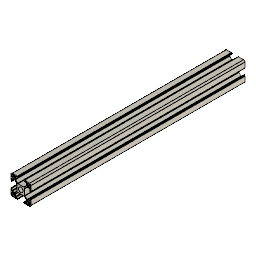
3030_Extrusion_Y_F01 (Autodesk Fusion 360 design; units mm, degrees)
Autodesk Fusion 360 part; units mm, degrees
sketch "スケッチ1" plane through (0, 0, 0) normal (0, 1, 0) x (1, 0, 0)
  line L0 (13, -15) -> (-13, -15)
  line L1 (-15, -13) -> (-15, 13)
  line L2 (-13, 15) -> (13, 15)
  line L3 (15, 13) -> (15, -13)
  line L4 (15, -15) -> (-15, 15) construction
  line L5 (-15, -15) -> (15, 15) construction
  circle A0 centre (0, 0) radius 3.4
  line L6 (-5.2, -15) -> (-5.2, -14.25)
  line L7 (-5.2, -14.25) -> (-4.2, -14.25)
  line L8 (-4.2, -14.25) -> (-4.2, -13.5)
  line L9 (-4.2, -13.5) -> (-7.75, -13.5)
  line L10 (-8.25, -13) -> (-8.25, -9.5178)
  line L11 (-8.1036, -9.1642) -> (-4.8858, -5.9464)
  line L12 (-4.5322, -5.8) -> (0, -5.8)
  arc A1 (-8.25, -13) -> (-7.75, -13.5) centre (-7.75, -13) ccw
  arc A2 (-8.1036, -9.1642) -> (-8.25, -9.5178) centre (-7.75, -9.5178) ccw
  arc A3 (-4.5322, -5.8) -> (-4.8858, -5.9464) centre (-4.5322, -6.3) ccw
  line L13 (-13, -13.5) -> (-10, -13.5)
  line L14 (-9.5, -13) -> (-9.5, -10)
  line L15 (-10, -9.5) -> (-13, -9.5)
  line L16 (-13.5, -10) -> (-13.5, -13)
  arc A4 (-13.5, -13) -> (-13, -13.5) centre (-13, -13) ccw
  arc A5 (-10, -13.5) -> (-9.5, -13) centre (-10, -13) ccw
  arc A6 (-9.5, -10) -> (-10, -9.5) centre (-10, -10) ccw
  arc A7 (-13, -9.5) -> (-13.5, -10) centre (-13, -10) ccw
  arc A8 (-15, -13) -> (-13, -15) centre (-13, -13) ccw
  arc A9 (-13, 15) -> (-15, 13) centre (-13, 13) ccw
  arc A10 (15, 13) -> (13, 15) centre (13, 13) ccw
  arc A11 (13, -15) -> (15, -13) centre (13, -13) ccw
  line L17 (0, 0) -> (0, -15) construction
  line L18 (5.2, -15) -> (5.2, -14.25)
  line L19 (5.2, -14.25) -> (4.2, -14.25)
  line L20 (4.2, -14.25) -> (4.2, -13.5)
  line L21 (4.2, -13.5) -> (7.75, -13.5)
  arc A12 (7.75, -13.5) -> (8.25, -13) centre (7.75, -13) ccw
  line L22 (8.25, -13) -> (8.25, -9.5178)
  arc A13 (8.25, -9.5178) -> (8.1036, -9.1642) centre (7.75, -9.5178) ccw
  line L23 (8.1036, -9.1642) -> (4.8858, -5.9464)
  arc A14 (4.8858, -5.9464) -> (4.5322, -5.8) centre (4.5322, -6.3) ccw
  line L24 (4.5322, -5.8) -> (0, -5.8)
  line L25 (15, -5.2) -> (14.25, -5.2)
  line L26 (14.25, -5.2) -> (14.25, -4.2)
  line L27 (14.25, -4.2) -> (13.5, -4.2)
  line L28 (13.5, -4.2) -> (13.5, -7.75)
  arc A15 (13, -8.25) -> (13.5, -7.75) centre (13, -7.75) ccw
  line L29 (13, -8.25) -> (9.5178, -8.25)
  arc A16 (9.1642, -8.1036) -> (9.5178, -8.25) centre (9.5178, -7.75) ccw
  line L30 (9.1642, -8.1036) -> (5.9464, -4.8858)
  arc A17 (5.8, -4.5322) -> (5.9464, -4.8858) centre (6.3, -4.5322) ccw
  line L31 (5.8, -4.5322) -> (5.8, 0)
  line L32 (5.8, 4.5322) -> (5.8, 0)
  arc A18 (5.9464, 4.8858) -> (5.8, 4.5322) centre (6.3, 4.5322) ccw
  line L33 (9.1642, 8.1036) -> (5.9464, 4.8858)
  arc A19 (9.5178, 8.25) -> (9.1642, 8.1036) centre (9.5178, 7.75) ccw
  line L34 (13, 8.25) -> (9.5178, 8.25)
  arc A20 (13.5, 7.75) -> (13, 8.25) centre (13, 7.75) ccw
  line L35 (13.5, 4.2) -> (13.5, 7.75)
  line L36 (14.25, 4.2) -> (13.5, 4.2)
  line L37 (14.25, 5.2) -> (14.25, 4.2)
  line L38 (15, 5.2) -> (14.25, 5.2)
  line L39 (13.5, -13) -> (13.5, -10)
  arc A21 (13.5, -10) -> (13, -9.5) centre (13, -10) ccw
  line L40 (13, -9.5) -> (10, -9.5)
  arc A22 (10, -9.5) -> (9.5, -10) centre (10, -10) ccw
  line L41 (9.5, -10) -> (9.5, -13)
  arc A23 (9.5, -13) -> (10, -13.5) centre (10, -13) ccw
  line L42 (10, -13.5) -> (13, -13.5)
  arc A24 (13, -13.5) -> (13.5, -13) centre (13, -13) ccw
  line L43 (5.2, 15) -> (5.2, 14.25)
  line L44 (5.2, 14.25) -> (4.2, 14.25)
  line L45 (4.2, 14.25) -> (4.2, 13.5)
  line L46 (4.2, 13.5) -> (7.75, 13.5)
  arc A25 (8.25, 13) -> (7.75, 13.5) centre (7.75, 13) ccw
  line L47 (8.25, 13) -> (8.25, 9.5178)
  arc A26 (8.1036, 9.1642) -> (8.25, 9.5178) centre (7.75, 9.5178) ccw
  line L48 (8.1036, 9.1642) -> (4.8858, 5.9464)
  arc A27 (4.5322, 5.8) -> (4.8858, 5.9464) centre (4.5322, 6.3) ccw
  line L49 (4.5322, 5.8) -> (0, 5.8)
  line L50 (-4.5322, 5.8) -> (0, 5.8)
  arc A28 (-4.8858, 5.9464) -> (-4.5322, 5.8) centre (-4.5322, 6.3) ccw
  line L51 (-8.1036, 9.1642) -> (-4.8858, 5.9464)
  arc A29 (-8.25, 9.5178) -> (-8.1036, 9.1642) centre (-7.75, 9.5178) ccw
  line L52 (-8.25, 13) -> (-8.25, 9.5178)
  arc A30 (-7.75, 13.5) -> (-8.25, 13) centre (-7.75, 13) ccw
  line L53 (-4.2, 13.5) -> (-7.75, 13.5)
  line L54 (-4.2, 14.25) -> (-4.2, 13.5)
  line L55 (-5.2, 14.25) -> (-4.2, 14.25)
  line L56 (-5.2, 15) -> (-5.2, 14.25)
  line L57 (13, 13.5) -> (10, 13.5)
  arc A31 (10, 13.5) -> (9.5, 13) centre (10, 13) ccw
  line L58 (9.5, 13) -> (9.5, 10)
  arc A32 (9.5, 10) -> (10, 9.5) centre (10, 10) ccw
  line L59 (10, 9.5) -> (13, 9.5)
  arc A33 (13, 9.5) -> (13.5, 10) centre (13, 10) ccw
  line L60 (13.5, 10) -> (13.5, 13)
  arc A34 (13.5, 13) -> (13, 13.5) centre (13, 13) ccw
  line L61 (-15, 5.2) -> (-14.25, 5.2)
  line L62 (-14.25, 5.2) -> (-14.25, 4.2)
  line L63 (-14.25, 4.2) -> (-13.5, 4.2)
  line L64 (-13.5, 4.2) -> (-13.5, 7.75)
  arc A35 (-13, 8.25) -> (-13.5, 7.75) centre (-13, 7.75) ccw
  line L65 (-13, 8.25) -> (-9.5178, 8.25)
  arc A36 (-9.1642, 8.1036) -> (-9.5178, 8.25) centre (-9.5178, 7.75) ccw
  line L66 (-9.1642, 8.1036) -> (-5.9464, 4.8858)
  arc A37 (-5.8, 4.5322) -> (-5.9464, 4.8858) centre (-6.3, 4.5322) ccw
  line L67 (-5.8, 4.5322) -> (-5.8, 0)
  line L68 (-5.8, -4.5322) -> (-5.8, 0)
  arc A38 (-5.9464, -4.8858) -> (-5.8, -4.5322) centre (-6.3, -4.5322) ccw
  line L69 (-9.1642, -8.1036) -> (-5.9464, -4.8858)
  arc A39 (-9.5178, -8.25) -> (-9.1642, -8.1036) centre (-9.5178, -7.75) ccw
  line L70 (-13, -8.25) -> (-9.5178, -8.25)
  arc A40 (-13.5, -7.75) -> (-13, -8.25) centre (-13, -7.75) ccw
  line L71 (-13.5, -4.2) -> (-13.5, -7.75)
  line L72 (-14.25, -4.2) -> (-13.5, -4.2)
  line L73 (-14.25, -5.2) -> (-14.25, -4.2)
  line L74 (-15, -5.2) -> (-14.25, -5.2)
  line L75 (-13.5, 13) -> (-13.5, 10)
  arc A41 (-13.5, 10) -> (-13, 9.5) centre (-13, 10) ccw
  line L76 (-13, 9.5) -> (-10, 9.5)
  arc A42 (-10, 9.5) -> (-9.5, 10) centre (-10, 10) ccw
  line L77 (-9.5, 10) -> (-9.5, 13)
  arc A43 (-9.5, 13) -> (-10, 13.5) centre (-10, 13) ccw
  line L78 (-10, 13.5) -> (-13, 13.5)
  arc A44 (-13, 13.5) -> (-13.5, 13) centre (-13, 13) ccw
  dimension "d1" = 30
  dimension "d2" = 30
  dimension "d3" = 6.8
  dimension "d4" = 1
  dimension "d5" = 0.75
  dimension "d6" = 0.75
  dimension "d7" = 4.2
  dimension "d8" = 8.25
  dimension "d9" = 0.75
  dimension "d10" = 9.2
  dimension "d13" = 0.5
  dimension "d14" = 0.5
  dimension "d15" = 0.5
  dimension "d16" = 4
  dimension "d17" = 1.5
  dimension "d18" = 0.5
  dimension "d19" = 0.5
  dimension "d20" = 4
  dimension "d21" = 2
  dimension "d23" = 360
  measures "d3" diameter of A0
  measures "d7" distance of A0.centre L8
  measures "d8" distance of A0.centre L10
  measures "d9" distance of L5 L11
  measures "d10" distance of L0 L12
  measures "d13" radius of A1
  measures "d14" radius of A2
  measures "d15" radius of A3
  measures "d17" distance of L0 L13
  measures "d18" radius of A4
  measures "d19" radius of A5
  measures "d20" distance of L13 L15
  measures "d21" radius of A8
extrude "押し出し1" add sketch "スケッチ1" along normal mid plane 320 contours L0 L1 L2 L3 L6 L7 L8 L9 L10 L11 L12 A1 A2 A3 A8 A9 A10 A11 L18 L19 L20 L21 A12 L22 A13 L23 A14 L24 L25 L26 L27 L28 A15 L29 A16 L30 A17 L31 L32 A18 L33 A19 L34 A20 L35 L36 L37 L38 L43 L44 L45 L46 A25 L47 A26 L48 A27 L49 L50 A28 L51 A29 L52 A30 L53 L54 L55 L56 L61 L62 L63 L64 A35 L65 A36 L66 A37 L67 L68 A38 L69 A39 L70 A40 L71 L72 L73 L74
